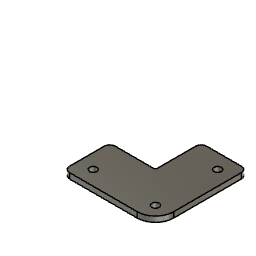
StandFront (Autodesk Fusion 360 design; units mm, degrees)
Autodesk Fusion 360 part; units mm, degrees
sketch "Sketch1" plane through (0, 0, 0) normal (0, 0, 1) x (1, 0, 0)
  line L0 (0, 0) -> (50, 0)
  line L1 (50, 0) -> (50, 50)
  line L2 (50, 50) -> (25, 50)
  line L3 (25, 50) -> (25, 25)
  line L4 (25, 25) -> (0, 25)
  line L5 (0, 25) -> (0, 0)
  line L6 (-25, 0) -> (-25, 55) construction
  dimension "d1" = 25
  dimension "d2" = 25
  dimension "d3" = 50
  dimension "d4" = 50
  constraint coincident L0.start L5.end
  constraint horizontal L0
  constraint perpendicular L0 L1
  constraint perpendicular L1 L2
  constraint perpendicular L2 L3
  constraint perpendicular L3 L4
  constraint perpendicular L0 L5
  constraint vertical L6
  measures "d1" distance of L4.end L0.start
  measures "d2" distance of L1.end L2.end
  measures "d3" distance of L0.start L0.end
  measures "d4" distance of L0.end L1.end
extrude "Extrude1" add sketch "Sketch1" along normal blind 3
ref_plane "WorkPlane1" through (-30, 0, 0) normal (1, 0, 0) x (0, 1, 0)
sketch "Sketch2" plane through (0, 0, 3) normal (0, 0, 1) x (-1, 0, 0)
  line L0 (0, -25) -> (0, 0)
  line L1 (0, 0) -> (-50, 0)
  line L2 (-50, 0) -> (-50, -50)
  line L3 (-50, -50) -> (-25, -50)
  line L4 (-25, -50) -> (-25, -25)
  line L5 (-25, -25) -> (0, -25)
  line L6 (-100, -100) -> (-70, -100)
  line L7 (-70, -100) -> (-70, -175)
  line L8 (-70, -175) -> (-100, -175)
  line L9 (-100, -175) -> (-100, -100)
  dimension "d10" = 30
  dimension "d11" = 75
  constraint horizontal L6
  constraint perpendicular L6 L7
  constraint perpendicular L7 L8
  constraint perpendicular L6 L9
  measures "d10" distance of L7.end L8.end
  measures "d11" distance of L6.end L7.end
fillet "Fillet1" radius 10 1 edges at (50, 0, 1.5)
fillet "Fillet2" radius 1 1 edges at (25, 25, 1.5)
fillet "Fillet3" radius 3 1 edges at (50, 50, 1.5)
fillet "Fillet4" radius 3 1 edges at (25, 50, 1.5)
fillet "Fillet5" radius 3 1 edges at (0, 25, 1.5)
fillet "Fillet6" radius 3 1 edges at (0, 0, 1.5)
sketch "Sketch5" plane through (0, 0, 3) normal (0, 0, 1) x (-1, 0, 0)
  arc A0 (0, -3) -> (-3, 0) centre (-3, -3) ccw
  line L0 (-3, 0) -> (-40, 0)
  arc A1 (-40, 0) -> (-50, -10) centre (-40, -10) ccw
  line L1 (-50, -10) -> (-50, -47)
  arc A2 (-50, -47) -> (-47, -50) centre (-47, -47) ccw
  line L2 (-47, -50) -> (-28, -50)
  arc A3 (-28, -50) -> (-25, -47) centre (-28, -47) ccw
  line L3 (-25, -47) -> (-25, -26)
  arc A4 (-24, -25) -> (-25, -26) centre (-24, -26) ccw
  line L4 (-24, -25) -> (-3, -25)
  arc A5 (-3, -25) -> (0, -22) centre (-3, -22) ccw
  line L5 (0, -22) -> (0, -3)
  circle A6 centre (-42, -8) radius 2
  circle A7 centre (-42, -42) radius 2
  circle A8 centre (-8, -8) radius 2
  dimension "d57" = 4
  dimension "d58" = 4
  dimension "d59" = 4
  dimension "d60" = 8
  dimension "d61" = 8
  dimension "d62" = 8
  dimension "d63" = 8
  dimension "d64" = 8
  dimension "d65" = 8
  measures "d57" diameter of A7
  measures "d58" diameter of A8
  measures "d59" diameter of A6
  measures "d60" distance of L5 A8.centre
  measures "d61" distance of L0 A8.centre
  measures "d62" distance of L1 A6.centre
  measures "d63" distance of L0 A6.centre
  measures "d64" distance of L2 A7.centre
  measures "d65" distance of L1 A7.centre
extrude "Extrude7" cut sketch "Sketch5" against normal blind 3 contours A6 | A7 | A8
